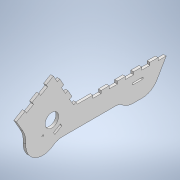
# Autodesk Inventor part: wooden_side
Saved by Autodesk Inventor 2020 (Build 240168000, 168)
## iProperties
Created: 2019-07-24
Part Number: wooden_side
Material: Generic
Document SubType Name: Modeling
Designer: erwin
Density: 1 g/cm^3
Appearance: Default
Author: erwin
Autodesk Inventor part; units mm, degrees
ref_plane "YZ Plane" through (0, 0, 0) normal (1, 0, 0) x (0, 1, 0)
ref_plane "XZ Plane" through (0, 0, 0) normal (0, 1, 0) x (-1, 0, 0)
ref_plane "XY Plane" through (0, 0, 0) normal (0, 0, 1) x (1, 0, 0)
sketch "Sketch1" plane through (0, 0, 0) normal (1, 0, 0) x (0, 1, 0)
  circle A0 centre (0, 316.1768) radius 4
  line L0 (0, -83.8232) -> (0, -123.8232)
  line L1 (-4, -83.8232) -> (-4, -123.8232)
  line L2 (4, -123.8232) -> (4, -83.8232)
  arc A1 (4, -83.8232) -> (-4, -83.8232) centre (0, -83.8232) ccw
  arc A2 (-4, -123.8232) -> (4, -123.8232) centre (0, -123.8232) ccw
  arc A3 (29.4615, 385.1479) -> (-59.8687, 271.0022) centre (0, 316.1768) ccw construction
  line L3 (-75, -123.8232) -> (-75, -83.8232) construction
  line L4 (45, -142.4909) -> (45, -229.6533) construction
  arc A4 (-75, -123.8232) -> (-37.5, -188.7751) centre (0, -123.8232) ccw construction
  circle A5 centre (0, 316.1768) radius 115 construction
  line L5 (-115, -63.8232) -> (-115, -123.8232) construction
  arc A6 (-115, -123.8232) -> (115, -123.8232) centre (0, -123.8232) ccw construction
  line L6 (115, -123.8232) -> (115, -63.8232) construction
  arc A7 (115, -63.8232) -> (-115, -63.8232) centre (0, -83.8232) ccw construction
  line L7 (111.5189, 432.5238) -> (211.5189, 259.3187)
  line L8 (211.5189, 259.3187) -> (45, 163.179)
  circle A8 centre (0, 316.1768) radius 45 construction
  arc A9 (29.4615, 385.1479) -> (-59.8687, 271.0022) centre (0, 316.1768) ccw
  line L9 (-75, -123.8232) -> (-75, -83.8232)
  arc A10 (-57.0417, -35.1278) -> (-75, -83.8232) centre (0, -83.8232) ccw
  arc A11 (-75, -123.8232) -> (-37.5, -188.7751) centre (0, -123.8232) ccw
  line L10 (-46.3992, 230.789) -> (-46.3992, -6.2697)
  arc A12 (-46.3992, 230.789) -> (-59.8687, 271.0022) centre (-113.1622, 230.789) ccw
  arc A13 (-57.0417, -35.1278) -> (-46.3992, -6.2697) centre (-90.846, -6.2697) ccw
  line L11 (45, -229.4783) -> (45, 163.179)
  line L12 (43.5102, 150.8148) -> (13.9439, 202.0253) construction
  line L13 (-38.9711, 293.6768) -> (-61.4711, 332.6479) construction
  line L14 (-61.4711, 332.6479) -> (-22.5, 355.1479) construction
  line L15 (29.4615, 385.1479) -> (111.5189, 432.5238)
  line L16 (45, -229.4783) -> (33, -229.4783)
  line L17 (33, -229.4783) -> (-37.5, -188.7751)
  line L18 (45, 316.1768) -> (45, 281.1768) construction
  line L19 (-75, -123.8232) -> (-75, -83.8232) construction
  arc A14 (75, -83.8232) -> (-75, -83.8232) centre (0, -83.8232) ccw construction
  line L20 (75, -83.8232) -> (75, -123.8232) construction
  arc A15 (-75, -123.8232) -> (75, -123.8232) centre (0, -123.8232) ccw construction
  point P0 (0, 0)
  point P1 (0, -103.8232)
  dimension "d7" = 230
  dimension "d0" = 8
  dimension "d1" = 8
  dimension "d2" = 400
  dimension "d3" = 40
  dimension "d5" = 150
  dimension "d8" = 115
  dimension "d9" = 200
  dimension "d10" = 200
  dimension "d12" = 90
  dimension "d13" = 12
  dimension "d15" = 120
  dimension "d16" = 120
  dimension "d17" = 75
  constraints: 44 end point, 32 point on circle, 15 centre point, 13 tangent, 10 parallel, 4 vertical, 2 coincident, 2 perpendicular, 1 collinear, 1 concentric, 1 midpoint, 1 point on line, 7 other
  measures "d0" diameter of A0
  measures "d1" diameter of A2
  measures "d2" distance of A0.centre L0.start
  measures "d3" distance of L0.start L0.end
  measures "d5" diameter of A3
  measures "d8" radius of A6
  measures "d9" distance of L7.end L12.start
  measures "d10" distance of L7.start L7.end
  measures "d12" diameter of A8
  measures "d13" distance of L11.start L16.end
  measures "d15" angle of L4 L17
  measures "d16" angle of L8 L11
  measures "d17" radius of A14
extrude "Extrusion1" add sketch "Sketch1" along normal blind 12
fillet "Fillet1" radius 100 1 edges at (6, 29.4615, 385.1479)
sketch "Sketch2" plane through (12, 0, 0) normal (1, 0, 0) x (0, 0, -1)
  line L0 (229.4783, 45) -> (-163.179, 45) construction
  line L1 (229.4783, 45) -> (193.4783, 45)
  line L2 (193.4783, 45) -> (193.4783, 33)
  line L3 (193.4783, 33) -> (229.4783, 33)
  line L4 (229.4783, 33) -> (229.4783, 45)
  line L5 (-163.179, 45) -> (-259.3187, 211.5189) construction
  line L6 (-432.5238, 111.5189) -> (-404.1377, 62.3528) construction
  line L7 (-259.3187, 211.5189) -> (-432.5238, 111.5189) construction
  line L8 (-432.5238, 111.5189) -> (-332.5238, -61.6862) construction
  line L9 (-332.5238, -61.6862) -> (-159.3187, 38.3138) construction
  line L10 (-159.3187, 38.3138) -> (-259.3187, 211.5189) construction
  line L11 (-259.3187, 211.5189) -> (-241.3187, 180.342)
  line L12 (-241.3187, 180.342) -> (-251.711, 174.342)
  line L13 (-251.711, 174.342) -> (-269.711, 205.5189)
  line L14 (-269.711, 205.5189) -> (-259.3187, 211.5189)
  line L15 (-432.5238, 111.5189) -> (-159.3187, 38.3138) construction
  line L16 (193.4783, 45) -> (157.4783, 45)
  line L17 (157.4783, 33) -> (193.4783, 33)
  line L18 (193.4783, 33) -> (193.4783, 45)
  line L19 (157.4783, 45) -> (157.4783, 33)
  line L20 (157.4783, 45) -> (121.4783, 45)
  line L21 (121.4783, 33) -> (157.4783, 33)
  line L22 (157.4783, 33) -> (157.4783, 45)
  line L23 (121.4783, 45) -> (121.4783, 33)
  line L24 (121.4783, 45) -> (85.4783, 45)
  line L25 (85.4783, 33) -> (121.4783, 33)
  line L26 (121.4783, 33) -> (121.4783, 45)
  line L27 (85.4783, 45) -> (85.4783, 33)
  line L28 (85.4783, 45) -> (49.4783, 45)
  line L29 (49.4783, 33) -> (85.4783, 33)
  line L30 (85.4783, 33) -> (85.4783, 45)
  line L31 (49.4783, 45) -> (49.4783, 33)
  line L32 (49.4783, 45) -> (13.4783, 45)
  line L33 (13.4783, 33) -> (49.4783, 33)
  line L34 (49.4783, 33) -> (49.4783, 45)
  line L35 (13.4783, 45) -> (13.4783, 33)
  line L36 (13.4783, 45) -> (-22.5217, 45)
  line L37 (-22.5217, 33) -> (13.4783, 33)
  line L38 (13.4783, 33) -> (13.4783, 45)
  line L39 (-22.5217, 45) -> (-22.5217, 33)
  line L40 (-22.5217, 45) -> (-58.5217, 45)
  line L41 (-58.5217, 33) -> (-22.5217, 33)
  line L42 (-22.5217, 33) -> (-22.5217, 45)
  line L43 (-58.5217, 45) -> (-58.5217, 33)
  line L44 (-58.5217, 45) -> (-94.5217, 45)
  line L45 (-94.5217, 33) -> (-58.5217, 33)
  line L46 (-58.5217, 33) -> (-58.5217, 45)
  line L47 (-94.5217, 45) -> (-94.5217, 33)
  line L48 (-94.5217, 45) -> (-130.5217, 45)
  line L49 (-130.5217, 33) -> (-94.5217, 33)
  line L50 (-94.5217, 33) -> (-94.5217, 45)
  line L51 (-130.5217, 45) -> (-130.5217, 33)
  line L52 (-130.5217, 45) -> (-166.5217, 45)
  line L53 (-166.5217, 33) -> (-130.5217, 33)
  line L54 (-130.5217, 33) -> (-130.5217, 45)
  line L55 (-166.5217, 45) -> (-166.5217, 33)
  line L56 (-166.5217, 45) -> (-202.5217, 45)
  line L57 (-202.5217, 33) -> (-166.5217, 33)
  line L58 (-166.5217, 33) -> (-166.5217, 45)
  line L59 (-202.5217, 45) -> (-202.5217, 33)
  line L60 (-251.711, 174.342) -> (-241.3187, 180.342)
  line L61 (-233.711, 143.1651) -> (-251.711, 174.342)
  line L62 (-241.3187, 180.342) -> (-223.3187, 149.1651)
  line L63 (-223.3187, 149.1651) -> (-233.711, 143.1651)
  line L64 (-233.711, 143.1651) -> (-223.3187, 149.1651)
  line L65 (-215.711, 111.9882) -> (-233.711, 143.1651)
  line L66 (-223.3187, 149.1651) -> (-205.3187, 117.9882)
  line L67 (-205.3187, 117.9882) -> (-215.711, 111.9882)
  line L68 (-215.711, 111.9882) -> (-205.3187, 117.9882)
  line L69 (-197.711, 80.8112) -> (-215.711, 111.9882)
  line L70 (-205.3187, 117.9882) -> (-187.3187, 86.8112)
  line L71 (-187.3187, 86.8112) -> (-197.711, 80.8112)
  line L72 (-197.711, 80.8112) -> (-187.3187, 86.8112)
  line L73 (-179.711, 49.6343) -> (-197.711, 80.8112)
  line L74 (-187.3187, 86.8112) -> (-169.3187, 55.6343)
  line L75 (-169.3187, 55.6343) -> (-179.711, 49.6343)
  line L76 (-259.3187, 211.5189) -> (-432.5238, 111.5189) projected
  line L77 (-269.711, 205.5189) -> (-300.8879, 187.5189)
  line L78 (-300.8879, 187.5189) -> (-294.8879, 177.1266)
  line L79 (-294.8879, 177.1266) -> (-263.711, 195.1266)
  line L80 (-263.711, 195.1266) -> (-269.711, 205.5189)
  line L81 (-294.8879, 177.1266) -> (-300.8879, 187.5189)
  line L82 (-326.0648, 159.1266) -> (-294.8879, 177.1266)
  line L83 (-300.8879, 187.5189) -> (-332.0648, 169.5189)
  line L84 (-332.0648, 169.5189) -> (-326.0648, 159.1266)
  line L85 (-290.4956, 193.5189) -> (-463.7007, 93.5189) construction
  line L86 (-326.0648, 159.1266) -> (-332.0648, 169.5189)
  line L87 (-357.2417, 141.1266) -> (-326.0648, 159.1266)
  line L88 (-332.0648, 169.5189) -> (-363.2417, 151.5189)
  line L89 (-363.2417, 151.5189) -> (-357.2417, 141.1266)
  line L90 (-321.6725, 175.5189) -> (-494.8776, 75.5189) construction
  line L91 (-357.2417, 141.1266) -> (-363.2417, 151.5189)
  line L92 (-388.4187, 123.1266) -> (-357.2417, 141.1266)
  line L93 (-363.2417, 151.5189) -> (-394.4187, 133.5189)
  line L94 (-394.4187, 133.5189) -> (-388.4187, 123.1266)
  line L95 (-352.8494, 157.5189) -> (-526.0545, 57.5189) construction
  line L96 (-388.4187, 123.1266) -> (-394.4187, 133.5189)
  line L97 (-419.5956, 105.1266) -> (-388.4187, 123.1266)
  line L98 (-394.4187, 133.5189) -> (-425.5956, 115.5189)
  line L99 (-425.5956, 115.5189) -> (-419.5956, 105.1266)
  line L100 (-384.0264, 139.5189) -> (-557.2314, 39.5189) construction
  line L101 (-232.0648, -3.6862) -> (-263.2417, -21.6862)
  line L102 (-263.2417, -21.6862) -> (-269.2417, -11.2939)
  line L103 (-269.2417, -11.2939) -> (-238.0648, 6.7061)
  line L104 (-238.0648, 6.7061) -> (-232.0648, -3.6862)
  circle A0 centre (-276.1768, 40) radius 30
  circle A1 centre (-316.1768, 0) radius 4 projected
  point P0 (-295.9212, 74.9164)
  dimension "d21" = 12
  dimension "d22" = 36
  dimension "d26" = 200
  dimension "d27" = 12
  dimension "d28" = 36
  dimension "d31" = 36
  dimension "d38" = 36
  dimension "d45" = 12
  dimension "d46" = 36
  dimension "d49" = 36
  dimension "d54" = 60
  dimension "d55" = 40
  dimension "d56" = 40
  dimension "d57" = 12
  constraints: 202 end point, 10 parallel, 6 perpendicular, 4 collinear, 4 point on line, 2 horizontal, 1 centre point, 1 midpoint, 164 other
  measures "d21" distance of L3.end L0.start
  measures "d22" distance of L2.end L3.end
  measures "d26" distance of L6.start L8.end
  measures "d27" distance of L11.end L12.end
  measures "d28" distance of L12.end L13.end
  measures "d31" distance of L2.end L17.start
  measures "d38" distance of L13.end L60.start
  measures "d45" distance of L77.end L78.end
  measures "d46" distance of L78.end L79.end
  measures "d49" distance of L13.end L81.end
  measures "d54" diameter of A0
  measures "d55" horizontal distance of A1.centre A0.centre
  measures "d56" horizontal distance of A1.centre A0.centre
  measures "d57" distance of L103.end L101.start
extrude "Extrusion2" cut sketch "Sketch2" against normal blind 12 contours L4 L3 L2 L1 | L19 L21 L23 L20 | L27 L29 L31 L28 | L35 L37 L39 L36 | L43 L45 L47 L44 | L11 L12 L13 L14 | L66 L67 L65 L63 | L78 L82 L84 L76 | L74 L75 L73 L71 | L89 L92 L94 L76 | L101 L102 L103 L104 | A0
equation "\"d8\" = 0.5 * d7"
equation "\"wood_thickness\" = 12"
body "Solid1"
